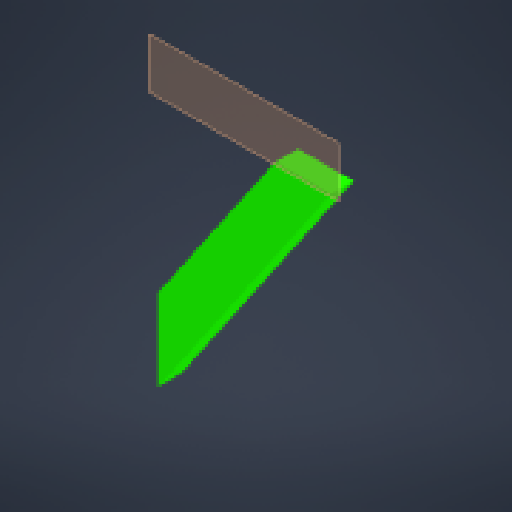
# Autodesk Inventor part: Top of head diagonals
Saved by Autodesk Inventor 2027 (Build 310192000, 192)
## iProperties
Created: 2026-05-29
Part Number: Top of head diagonals
Material: Generic
Document SubType Name: Modeling
Designer: lucas
Density: 1 g/cm^3
Appearance: Default
Author: lucas
Autodesk Inventor part; units mm, degrees
ref_plane "YZ Plane" through (0, 0, 0) normal (1, 0, 0) x (0, 1, 0)
ref_plane "XZ Plane" through (0, 0, 0) normal (0, 1, 0) x (-1, 0, 0)
ref_plane "XY Plane" through (0, 0, 0) normal (0, 0, 1) x (1, 0, 0)
ref_plane "Work Plane1" through (0, 0, 0) normal (0, 0, 1) x (1, 0, 0)
sketch "Sketch1" plane through (0, 0, 0) normal (0, 0, 1) x (1, 0, 0)
  line L0 (-190.5, -50.8) -> (190.5, -50.8) projected
  line L1 (-190.5, -609.6) -> (-190.5, -508) projected
  line L2 (190.5, -50.8) -> (-190.5, -609.6)
  line L3 (-190.5, -508) -> (-190.5, 1727.2) projected
  line L4 (-37.5923, -204.9815) -> (-190.5, -429.2461)
  line L5 (-37.5923, -204.9815) -> (67.5314, -50.8)
  line L6 (190.5, -50.8) -> (67.5314, -50.8)
  line L7 (-190.5, -429.2461) -> (-190.5, -609.6)
  point P0 (0, 0)
  point P1 (-190.5, -429.2461)
  dimension "d0" = 101.6
  constraints: 10 end point, 1 collinear, 1 point on line, 1 vertical
  measures "d0" distance between parallel lines of L2 L4
extrude "Extrusion1" add sketch "Sketch1" against normal blind 50.8 contours L0 L2 L1 L3 L4 L5
body "Solid1"
